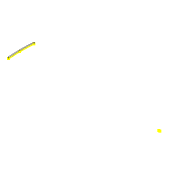
# Autodesk Inventor part: Part_5
Saved by Autodesk Inventor 2022 (Build 260153000, 153)
## iProperties
Created: 2022-04-26
Part Number: Part_5
Material: Generic
Document SubType Name: Modeling
Designer: dell
Density: 1 g/cm^3
Appearance: Default
Author: dell
Autodesk Inventor part; units mm, degrees
ref_plane "YZ Plane" through (0, 0, 0) normal (1, 0, 0) x (0, 1, 0)
ref_plane "XZ Plane" through (0, 0, 0) normal (0, 1, 0) x (-1, 0, 0)
ref_plane "XY Plane" through (0, 0, 0) normal (0, 0, 1) x (1, 0, 0)
sketch "Sketch1" plane through (0, 0, 0) normal (0, 1, 0) x (-1, 0, 0)
  line L0 (0, 0) -> (0, -183.747) construction
  line L1 (-3, 0) -> (-3, -183.747)
  line L2 (3, -183.747) -> (3, 0)
  arc A0 (3, 0) -> (-3, 0) centre (0, 0) ccw
  arc A1 (-3, -183.747) -> (3, -183.747) centre (0, -183.747) ccw
  circle A2 centre (0, 0) radius 1.5
  circle A3 centre (0, -183.747) radius 1.5
  circle A4 centre (0, -81.332) radius 1.5
  arc A5 (3, -183.747) -> (3, 0) centre (-992.7707, -91.8735) ccw
  arc A6 (-3, -183.747) -> (-3, 0) centre (-998.7707, -91.8735) ccw
  circle A7 centre (4.2, -84.209) radius 1.5
  point P0 (0, -91.8735)
  dimension "d0" = 183.747
  dimension "d1" = 6
  dimension "d2" = 3
  dimension "d3" = 3
  dimension "d8" = 3
  dimension "d9" = 81.332
  dimension "d12" = 1000
  dimension "d13" = 1000
  dimension "d14" = 3
  dimension "d15" = 4.2
  constraints: 8 centre point, 8 end point, 8 point on circle, 4 tangent, 2 coincident, 1 midpoint, 1 parallel, 1 point on line, 1 vertical
  measures "d0" distance of L0.start L0.end
  measures "d1" diameter of A1
  measures "d2" diameter of A2
  measures "d3" diameter of A3
  measures "d8" diameter of A4
  measures "d9" distance of L0.start A4.centre
  measures "d12" radius of A6
  measures "d13" radius of A5
  measures "d14" diameter of A7
  measures "d15" distance from line of L0 A7.centre
extrude "Extrusion1" add sketch "Sketch1" along normal blind 8 contours A0 L2 A7 A1 A6 A4 | A5 L2 A7 | A4 A6 picked at (1.2824, -81.3237)
sketch "Sketch2" plane through (0, 0, 0) normal (0, -1, 0) x (1, 0, 0)
  arc A0 (3, 0) -> (-3, 0) centre (0, 0) ccw projected
  arc A1 (-3, 0) -> (-3, -183.747) centre (992.7707, -91.8735) ccw projected
  arc A2 (-3, -183.747) -> (3, -183.747) centre (0, -183.747) ccw projected
  arc A3 (3, 0) -> (3, -183.747) centre (998.7707, -91.8735) ccw projected
  circle A4 centre (-4.2, -84.209) radius 1.5 projected
  circle A5 centre (0, -183.747) radius 1.5 projected
  circle A6 centre (0, 0) radius 1.5 projected
body "Solid1"
